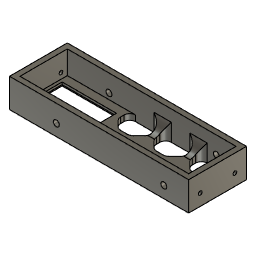
Grill_MAINS_Panels (Autodesk Fusion 360 design; units mm, degrees)
Autodesk Fusion 360 part; units mm, degrees
sketch "Skizze1" plane through (0, 0, 0) normal (0, 0, 1) x (1, 0, 0)
  line L0 (0, 0) -> (155, 0)
  line L1 (155, 0) -> (155, 50)
  line L2 (155, 50) -> (0, 50)
  line L3 (0, 50) -> (0, 0)
  dimension "d1" = 155
  dimension "d2" = 50
  constraint horizontal L0
  constraint vertical L1
  constraint horizontal L2
  constraint vertical L3
  constraint coincident L0.start L3.end
  measures "d1" distance of L0.start L0.end
  measures "d2" distance of L0.start L2.end
extrude "Extrusion1" add sketch "Skizze1" along normal blind 5
sketch "Skizze2" plane through (0, 0, 5) normal (0, 0, 1) x (-1, 0, 0)
  line L0 (0, -50) -> (0, 0)
  line L1 (0, 0) -> (-155, 0)
  line L2 (-155, 0) -> (-155, -50)
  line L3 (-155, -50) -> (0, -50)
  line L4 (-4.5, -45.5) -> (-150.5, -45.5)
  line L5 (-150.5, -45.5) -> (-150.5, -4.5)
  line L6 (-150.5, -4.5) -> (-4.5, -4.5)
  line L7 (-4.5, -4.5) -> (-4.5, -45.5)
  constraint horizontal L4
  constraint vertical L5
  constraint horizontal L6
  constraint vertical L7
extrude "Extrusion2" add sketch "Skizze2" along normal blind 20
sketch "Skizze3" plane through (0, 0, 5) normal (0, 0, 1) x (-1, 0, 0)
  line L0 (-150.5, -4.5) -> (-150.5, -45.5)
  line L1 (-4.5, -45.5) -> (-4.5, -4.5)
  line L2 (-4.5, -22.5) -> (-14.5, -22.5)
  line L3 (-4.5, -27.5) -> (-14.5, -27.5)
  line L4 (-22.5, -45.5) -> (-22.5, -35.5)
  line L5 (-22.5, -4.5) -> (-22.5, -14.5)
  line L6 (-14.5, -22.5) -> (-22.5, -14.5)
  line L7 (-14.5, -27.5) -> (-22.5, -35.5)
  line L8 (-22.5, -4.5) -> (-27.5, -4.5)
  line L9 (-27.5, -45.5) -> (-27.5, -35.5)
  line L10 (-27.5, -4.5) -> (-27.5, -14.5)
  line L11 (-27.5, -4.5) -> (-35.5, -4.5)
  line L12 (-35.5, -4.5) -> (-35.5, -22.5)
  line L13 (-27.5, -35.5) -> (-35.5, -27.5)
  line L14 (-27.5, -14.5) -> (-35.5, -22.5)
  line L15 (-35.5, -22.5) -> (-45.5, -22.5)
  line L16 (-35.5, -27.5) -> (-45.5, -27.5)
  line L17 (-35.5, -4.5) -> (-53.5, -4.5)
  line L18 (-53.5, -4.5) -> (-53.5, -14.5)
  line L19 (-45.5, -22.5) -> (-53.5, -14.5)
  line L20 (-53.5, -45.5) -> (-53.5, -35.5)
  line L21 (-53.5, -35.5) -> (-45.5, -27.5)
  line L22 (-53.5, -45.5) -> (-58.5, -45.5)
  line L23 (-58.5, -45.5) -> (-58.5, -35.5)
  line L24 (-53.5, -4.5) -> (-58.5, -4.5)
  line L25 (-58.5, -4.5) -> (-58.5, -14.5)
  line L26 (-58.5, -4.5) -> (-66.5, -4.5)
  line L27 (-66.5, -4.5) -> (-66.5, -22.5)
  line L28 (-58.5, -14.5) -> (-66.5, -22.5)
  line L29 (-66.5, -27.5) -> (-58.5, -35.5)
  line L30 (-66.5, -27.5) -> (-76.5, -27.5)
  line L31 (-66.5, -22.5) -> (-76.5, -22.5)
  line L32 (-76.5, -4.5) -> (-84.5, -4.5)
  line L33 (-84.5, -4.5) -> (-84.5, -14.5)
  line L34 (-84.5, -14.5) -> (-76.5, -22.5)
  line L35 (-76.5, -27.5) -> (-84.5, -35.5)
  line L36 (-84.5, -35.5) -> (-84.5, -45.5)
  line L37 (-84.5, -45.5) -> (-89.5, -45.5)
  line L38 (-89.5, -45.5) -> (-89.5, -35.5)
  line L39 (-89.5, -35.5) -> (-97.5, -27.5)
  line L40 (-89.5, -35.5) -> (-78.1863, -35.5) construction
  line L41 (-97.5, -27.5) -> (-107.5, -27.5)
  line L42 (-107.5, -27.5) -> (-115.5, -35.5)
  line L43 (-115.5, -35.5) -> (-115.5, -45.5)
  line L44 (-84.5, -4.5) -> (-89.5, -4.5)
  line L45 (-89.5, -4.5) -> (-89.5, -14.5)
  line L46 (-89.5, -14.5) -> (-97.5, -22.5)
  line L47 (-89.5, -14.5) -> (-78.1863, -14.5) construction
  line L48 (-97.5, -22.5) -> (-107.5, -22.5)
  line L49 (-107.5, -22.5) -> (-115.5, -14.5)
  line L50 (-115.5, -14.5) -> (-115.5, -4.5)
  line L51 (-115.5, -4.5) -> (-120.5, -4.5)
  line L52 (-120.5, -4.5) -> (-120.5, -14.5)
  line L53 (-120.5, -14.5) -> (-128.5, -22.5)
  line L54 (-120.5, -14.5) -> (-109.1863, -14.5) construction
  line L55 (-128.5, -22.5) -> (-138.5, -22.5)
  line L56 (-138.5, -22.5) -> (-146.5, -14.5)
  line L57 (-138.5, -22.5) -> (-127.1863, -22.5) construction
  line L58 (-146.5, -14.5) -> (-146.5, -4.5)
  line L59 (-138.5, -27.5) -> (-146.5, -35.5)
  line L60 (-146.5, -35.5) -> (-146.5, -45.5)
  line L61 (-138.5, -27.5) -> (-128.5, -27.5)
  line L62 (-128.5, -27.5) -> (-120.5, -35.5)
  line L63 (-128.5, -27.5) -> (-117.1863, -27.5) construction
  line L64 (-120.5, -35.5) -> (-120.5, -45.5)
  line L65 (-4.5, -27.5) -> (-4.5, -45.5)
  line L66 (-4.5, -45.5) -> (-22.5, -45.5)
  line L67 (-4.5, -22.5) -> (-4.5, -4.5)
  line L68 (-4.5, -4.5) -> (-22.5, -4.5)
  line L69 (-27.5, -4.5) -> (-53.5, -4.5)
  line L70 (-58.5, -4.5) -> (-84.5, -4.5)
  line L71 (-89.5, -4.5) -> (-115.5, -4.5)
  line L72 (-120.5, -4.5) -> (-146.5, -4.5)
  line L73 (-146.5, -45.5) -> (-120.5, -45.5)
  line L74 (-115.5, -45.5) -> (-89.5, -45.5)
  line L75 (-84.5, -45.5) -> (-58.5, -45.5)
  line L76 (-53.5, -45.5) -> (-27.5, -45.5)
  dimension "d13" = 10
  dimension "d14" = 10
  dimension "d15" = 18
  dimension "d16" = 10
  dimension "d17" = 18
  dimension "d18" = 10
  dimension "d19" = 5
  dimension "d20" = 5
  dimension "d21" = 10
  dimension "d22" = 10
  dimension "d23" = 8
  dimension "d24" = 18
  dimension "d25" = 5
  dimension "d26" = 10
  dimension "d27" = 10
  dimension "d28" = 18
  dimension "d29" = 10
  dimension "d30" = 10
  dimension "d31" = 5
  dimension "d32" = 10
  dimension "d33" = 5
  dimension "d34" = 10
  dimension "d35" = 8
  dimension "d36" = 18
  dimension "d37" = 5
  dimension "d38" = 10
  dimension "d39" = 10
  dimension "d40" = 8
  dimension "d41" = 10
  dimension "d42" = 5
  dimension "d43" = 10
  dimension "d44" = 135
  dimension "d45" = 10
  dimension "d46" = 5
  dimension "d47" = 10
  dimension "d48" = 135
  dimension "d49" = 10
  dimension "d50" = 5
  dimension "d51" = 10
  dimension "d52" = 135
  dimension "d53" = 10
  dimension "d54" = 135
  dimension "d56" = 10
  dimension "d57" = 45
  constraint perpendicular L1 L3
  constraint perpendicular L5 L8
  constraint perpendicular L8 L10
  constraint perpendicular L10 L11
  constraint perpendicular L11 L12
  constraint perpendicular L12 L17
  constraint perpendicular L17 L18
  constraint perpendicular L20 L22
  constraint perpendicular L18 L24
  constraint perpendicular L24 L25
  constraint perpendicular L25 L26
  constraint perpendicular L26 L27
  constraint perpendicular L28 L29
  constraint perpendicular L27 L31
  constraint perpendicular L32 L33
  constraint perpendicular L34 L35
  constraint perpendicular L36 L37
  constraint perpendicular L37 L38
  constraint horizontal L40
  constraint perpendicular L38 L41
  constraint perpendicular L39 L42
  constraint perpendicular L33 L44
  constraint perpendicular L44 L45
  constraint horizontal L47
  constraint perpendicular L46 L49
  constraint perpendicular L50 L51
  constraint horizontal L54
  constraint horizontal L57
  constraint horizontal L63
  constraint coincident L1.start L65.end
  constraint perpendicular L3 L65
  constraint perpendicular L65 L66
  constraint coincident L1.end L67.end
  constraint perpendicular L2 L67
  constraint perpendicular L5 L68
  constraint perpendicular L33 L70
  constraint perpendicular L50 L71
  constraint perpendicular L58 L72
  constraint perpendicular L64 L73
  constraint perpendicular L38 L74
  constraint perpendicular L23 L75
  constraint perpendicular L9 L76
  measures "d13" distance of L2.start L2.end
  measures "d14" distance of L3.start L3.end
  measures "d15" distance of L1.start L4.start
  measures "d16" distance of L4.start L4.end
  measures "d17" distance of L1.end L5.start
  measures "d18" distance of L5.start L5.end
  measures "d19" distance of L4.start L9.start
  measures "d20" distance of L5.start L8.end
  measures "d21" distance of L9.start L9.end
  measures "d22" distance of L8.end L10.end
  measures "d23" distance of L8.end L11.end
  measures "d24" distance of L11.end L12.end
  measures "d25" distance of L12.end L13.end
  measures "d26" distance of L12.end L15.end
  measures "d27" distance of L13.end L16.end
  measures "d28" distance of L11.end L17.end
  measures "d29" distance of L17.end L18.end
  measures "d30" distance of L20.start L20.end
  measures "d31" distance of L20.start L22.end
  measures "d32" distance of L22.end L23.end
  measures "d33" distance of L17.end L24.end
  measures "d34" distance of L24.end L25.end
  measures "d35" distance of L24.end L26.end
  measures "d36" distance of L26.end L27.end
  measures "d37" distance of L27.end L29.start
  measures "d38" distance of L29.start L30.end
  measures "d39" distance of L27.end L31.end
  measures "d40" distance of L32.start L32.end
  measures "d41" distance of L32.end L33.end
  measures "d42" distance of L36.end L37.end
  measures "d43" distance of L37.end L38.end
  measures "d44" angle of L39 L40
  measures "d45" distance of L39.end L41.end
  measures "d46" distance of L32.end L44.end
  measures "d47" distance of L44.end L45.end
  measures "d48" angle of L46 L47
  measures "d49" distance of L46.end L48.end
  measures "d50" distance of L50.end L51.end
  measures "d51" distance of L51.end L52.end
  measures "d52" angle of L53 L54
  measures "d53" distance of L53.end L55.end
  measures "d54" angle of L56 L57
  measures "d56" distance of L59.start L61.end
  measures "d57" angle of L62 L63
extrude "Extrusion3" cut sketch "Skizze3" against normal blind 5
fillet "Abrundung1" radius 5 56 edges at (22.5, 45.5, 2.5) (53.5, 45.5, 2.5) (84.5, 45.5, 2.5) (115.5, 45.5, 2.5) (146.5, 45.5, 2.5) (146.5, 35.5, 2.5) (120.5, 35.5, 2.5) (128.5, 27.5, 2.5) (138.5, 27.5, 2.5) (115.5, 35.5, 2.5) (107.5, 27.5, 2.5) (97.5, 27.5, 2.5) (89.5, 35.5, 2.5) (89.5, 45.5, 2.5) (120.5, 45.5, 2.5) (146.5, 14.5, 2.5) (138.5, 22.5, 2.5) (128.5, 22.5, 2.5) (120.5, 14.5, 2.5) (115.5, 14.5, 2.5) (107.5, 22.5, 2.5) (97.5, 22.5, 2.5) (89.5, 14.5, 2.5) (84.5, 35.5, 2.5) (84.5, 14.5, 2.5) (76.5, 22.5, 2.5) (76.5, 27.5, 2.5) (66.5, 27.5, 2.5) (66.5, 22.5, 2.5) (58.5, 14.5, 2.5) (58.5, 35.5, 2.5) (58.5, 45.5, 2.5) (53.5, 35.5, 2.5) (45.5, 27.5, 2.5) (45.5, 22.5, 2.5) (53.5, 14.5, 2.5) (35.5, 27.5, 2.5) (35.5, 22.5, 2.5) (27.5, 14.5, 2.5) (27.5, 35.5, 2.5) (27.5, 45.5, 2.5) (22.5, 35.5, 2.5) (14.5, 27.5, 2.5) (14.5, 22.5, 2.5) (22.5, 14.5, 2.5) (146.5, 4.5, 2.5) (120.5, 4.5, 2.5) (115.5, 4.5, 2.5) (84.5, 4.5, 2.5) (89.5, 4.5, 2.5) (58.5, 4.5, 2.5) (53.5, 4.5, 2.5) (27.5, 4.5, 2.5) (22.5, 4.5, 2.5) (4.5, 22.5, 2.5) (4.5, 27.5, 2.5)
fillet "Abrundung2" radius 10 5 edges at (25, 45.5, 5) (56, 45.5, 5) (87, 45.5, 5) (118, 45.5, 5) (146, 45.5, 5)
fillet "Abrundung3" radius 10 5 edges at (146, 4.5, 5) (118, 4.5, 5) (87, 4.5, 5) (56, 4.5, 5) (25, 4.5, 5)
extrude "Extrusion4" cut 1 faces at (53.1667, 48.5, 25) along direction (0, 0, -1) blind 5
hole "Bohrung1" at (0, 40, 10) direction (1, 0, 0) diameter 3.2 depth 10 tip angle 180
hole "Bohrung2" at (0, 10, 10) direction (1, 0, 0) diameter 3.2 depth 10 tip angle 180
hole "Bohrung3" at (40.5, 45.5, 10) direction (0, 1, 0) diameter 5.2 depth 10 tip angle 180
hole "Bohrung4" at (133.5, 45.5, 10) direction (0, 1, 0) diameter 5.2 depth 10 tip angle 180
hole "Bohrung5" at (133.5, 4.5, 10) direction (0, -1, 0) diameter 5.2 depth 10 tip angle 180
hole "Bohrung6" at (40.5, 4.5, 10) direction (0, -1, 0) diameter 5.2 depth 10 tip angle 180
delete_face "Fläche löschen1" 1 faces at (9.2621, 27.5057, 3.3333)
delete_face "Fläche löschen2" 1 faces at (9.2621, 22.4943, 3.3333)
delete_face "Fläche löschen3" 1 faces at (23.4001, 5.0158, 11.8299)
delete_face "Fläche löschen4" 1 faces at (26.8017, 45.2968, 12.9942)
sketch "Skizze4" plane through (0, 0, 5) normal (0, 0, 1) x (-1, 0, 0)
  line L0 (-22.5, -40.5) -> (-22.5, -37.5711)
  arc A0 (-21.0355, -34.0355) -> (-22.5, -37.5711) centre (-17.5, -37.5711) ccw
  line L1 (-21.0355, -34.0355) -> (-15.9645, -28.9645)
  arc A1 (-12.4289, -27.5) -> (-15.9645, -28.9645) centre (-12.4289, -32.5) ccw
  line L2 (-12.4289, -27.5) -> (-4.5, -27.5)
  line L3 (-4.5, -27.5) -> (-4.5, -22.5)
  line L4 (-4.5, -22.5) -> (-12.4289, -22.5)
  arc A2 (-15.9645, -21.0355) -> (-12.4289, -22.5) centre (-12.4289, -17.5) ccw
  line L5 (-15.9645, -21.0355) -> (-21.0355, -15.9645)
  arc A3 (-22.5, -12.4289) -> (-21.0355, -15.9645) centre (-17.5, -12.4289) ccw
  line L6 (-22.5, -12.4289) -> (-22.5, -9.5)
  arc A4 (-17.5, -4.5) -> (-22.5, -9.5) centre (-17.5, -9.5) ccw
  line L7 (-17.5, -4.5) -> (-32.5, -4.5)
  arc A5 (-27.5, -9.5) -> (-32.5, -4.5) centre (-32.5, -9.5) ccw
  line L8 (-27.5, -9.5) -> (-27.5, -12.4289)
  arc A6 (-28.9645, -15.9645) -> (-27.5, -12.4289) centre (-32.5, -12.4289) ccw
  line L9 (-28.9645, -15.9645) -> (-34.0355, -21.0355)
  arc A7 (-37.5711, -22.5) -> (-34.0355, -21.0355) centre (-37.5711, -17.5) ccw
  line L10 (-37.5711, -22.5) -> (-43.4289, -22.5)
  arc A8 (-46.9645, -21.0355) -> (-43.4289, -22.5) centre (-43.4289, -17.5) ccw
  line L11 (-46.9645, -21.0355) -> (-52.0355, -15.9645)
  arc A9 (-53.0509, -14.5) -> (-52.0355, -15.9645) centre (-48.5, -12.4289) ccw
  line L12 (-53.0509, -14.5) -> (-58.9491, -14.5)
  arc A10 (-59.9645, -15.9645) -> (-58.9491, -14.5) centre (-63.5, -12.4289) ccw
  line L13 (-59.9645, -15.9645) -> (-65.0355, -21.0355)
  arc A11 (-68.5711, -22.5) -> (-65.0355, -21.0355) centre (-68.5711, -17.5) ccw
  line L14 (-68.5711, -22.5) -> (-74.4289, -22.5)
  arc A12 (-77.9645, -21.0355) -> (-74.4289, -22.5) centre (-74.4289, -17.5) ccw
  line L15 (-77.9645, -21.0355) -> (-83.0355, -15.9645)
  arc A13 (-84.0509, -14.5) -> (-83.0355, -15.9645) centre (-79.5, -12.4289) ccw
  line L16 (-84.0509, -14.5) -> (-89.9491, -14.5)
  arc A14 (-90.9645, -15.9645) -> (-89.9491, -14.5) centre (-94.5, -12.4289) ccw
  line L17 (-90.9645, -15.9645) -> (-96.0355, -21.0355)
  arc A15 (-99.5711, -22.5) -> (-96.0355, -21.0355) centre (-99.5711, -17.5) ccw
  line L18 (-99.5711, -22.5) -> (-105.4289, -22.5)
  arc A16 (-108.9645, -21.0355) -> (-105.4289, -22.5) centre (-105.4289, -17.5) ccw
  line L19 (-108.9645, -21.0355) -> (-114.0355, -15.9645)
  arc A17 (-115.0509, -14.5) -> (-114.0355, -15.9645) centre (-110.5, -12.4289) ccw
  line L20 (-115.0509, -14.5) -> (-120.9491, -14.5)
  arc A18 (-121.9645, -15.9645) -> (-120.9491, -14.5) centre (-125.5, -12.4289) ccw
  line L21 (-121.9645, -15.9645) -> (-127.0355, -21.0355)
  arc A19 (-130.5711, -22.5) -> (-127.0355, -21.0355) centre (-130.5711, -17.5) ccw
  line L22 (-130.5711, -22.5) -> (-136.4289, -22.5)
  arc A20 (-139.9645, -21.0355) -> (-136.4289, -22.5) centre (-136.4289, -17.5) ccw
  line L23 (-139.9645, -21.0355) -> (-145.0355, -15.9645)
  arc A21 (-146.0509, -14.5) -> (-145.0355, -15.9645) centre (-141.5, -12.4289) ccw
  line L24 (-146.0509, -14.5) -> (-150.5, -14.5)
  line L25 (-150.5, -14.5) -> (-150.5, -35.5)
  line L26 (-150.5, -35.5) -> (-146.0509, -35.5)
  arc A22 (-145.0355, -34.0355) -> (-146.0509, -35.5) centre (-141.5, -37.5711) ccw
  line L27 (-145.0355, -34.0355) -> (-139.9645, -28.9645)
  arc A23 (-136.4289, -27.5) -> (-139.9645, -28.9645) centre (-136.4289, -32.5) ccw
  line L28 (-136.4289, -27.5) -> (-130.5711, -27.5)
  arc A24 (-127.0355, -28.9645) -> (-130.5711, -27.5) centre (-130.5711, -32.5) ccw
  line L29 (-127.0355, -28.9645) -> (-121.9645, -34.0355)
  arc A25 (-120.9491, -35.5) -> (-121.9645, -34.0355) centre (-125.5, -37.5711) ccw
  line L30 (-120.9491, -35.5) -> (-115.0509, -35.5)
  arc A26 (-114.0355, -34.0355) -> (-115.0509, -35.5) centre (-110.5, -37.5711) ccw
  line L31 (-114.0355, -34.0355) -> (-108.9645, -28.9645)
  arc A27 (-105.4289, -27.5) -> (-108.9645, -28.9645) centre (-105.4289, -32.5) ccw
  line L32 (-105.4289, -27.5) -> (-99.5711, -27.5)
  arc A28 (-96.0355, -28.9645) -> (-99.5711, -27.5) centre (-99.5711, -32.5) ccw
  line L33 (-96.0355, -28.9645) -> (-90.9645, -34.0355)
  arc A29 (-89.9491, -35.5) -> (-90.9645, -34.0355) centre (-94.5, -37.5711) ccw
  line L34 (-89.9491, -35.5) -> (-84.0509, -35.5)
  arc A30 (-83.0355, -34.0355) -> (-84.0509, -35.5) centre (-79.5, -37.5711) ccw
  line L35 (-83.0355, -34.0355) -> (-77.9645, -28.9645)
  arc A31 (-74.4289, -27.5) -> (-77.9645, -28.9645) centre (-74.4289, -32.5) ccw
  line L36 (-74.4289, -27.5) -> (-68.5711, -27.5)
  arc A32 (-65.0355, -28.9645) -> (-68.5711, -27.5) centre (-68.5711, -32.5) ccw
  line L37 (-65.0355, -28.9645) -> (-59.9645, -34.0355)
  arc A33 (-58.9491, -35.5) -> (-59.9645, -34.0355) centre (-63.5, -37.5711) ccw
  line L38 (-58.9491, -35.5) -> (-53.0509, -35.5)
  arc A34 (-52.0355, -34.0355) -> (-53.0509, -35.5) centre (-48.5, -37.5711) ccw
  line L39 (-52.0355, -34.0355) -> (-46.9645, -28.9645)
  arc A35 (-43.4289, -27.5) -> (-46.9645, -28.9645) centre (-43.4289, -32.5) ccw
  line L40 (-43.4289, -27.5) -> (-37.5711, -27.5)
  arc A36 (-34.0355, -28.9645) -> (-37.5711, -27.5) centre (-37.5711, -32.5) ccw
  line L41 (-34.0355, -28.9645) -> (-28.9645, -34.0355)
  arc A37 (-27.5, -37.5711) -> (-28.9645, -34.0355) centre (-32.5, -37.5711) ccw
  line L42 (-27.5, -37.5711) -> (-27.5, -40.5)
  arc A38 (-32.5, -45.5) -> (-27.5, -40.5) centre (-32.5, -40.5) ccw
  line L43 (-32.5, -45.5) -> (-17.5, -45.5)
  arc A39 (-22.5, -40.5) -> (-17.5, -45.5) centre (-17.5, -40.5) ccw
  line L44 (-4.5, -25) -> (-4.5, -45.5)
  line L45 (-4.5, -45.5) -> (-45.5, -45.5)
  line L46 (-45.5, -45.5) -> (-45.5, -4.5)
  line L47 (-45.5, -4.5) -> (-4.5, -4.5)
  line L48 (-4.5, -4.5) -> (-4.5, -45.5)
  dimension "d98" = 20.5
  dimension "d99" = 41
  dimension "d100" = 41
  constraint midpoint L3 L44.start
  constraint perpendicular L2 L44
  constraint horizontal L45
  constraint vertical L46
  constraint horizontal L47
  constraint vertical L48
  measures "d98" distance of L44.start L44.end
  measures "d99" distance of L44.end L45.end
  measures "d100" distance of L44.end L47.end
extrude "Extrusion5" add sketch "Skizze4" against normal blind 5 contours L0 A0 L1 A1 L2 A39 L44 L45 L48 | A35 L40 A36 L41 A37 L42 A38 L45 L46 | A5 L8 A6 L9 A7 L10 A8 L46 L47 | L4 A2 L5 A3 L6 A4 L47 L48
hole "Bohrung7" at (9, 41, 5) direction (0, 0, -1) diameter 3.2 depth 10 tip angle 180
hole "Bohrung8" at (9, 9, 5) direction (0, 0, -1) diameter 3.2 depth 10 tip angle 180
hole "Bohrung9" at (41, 41, 5) direction (0, 0, -1) diameter 3.2 depth 10 tip angle 180
hole "Bohrung10" at (41, 9, 5) direction (0, 0, -1) diameter 3.2 depth 10 tip angle 180
sketch "Skizze5" plane through (0, 0, 5) normal (0, 0, 1) x (-1, 0, 0)
  circle A0 centre (-41, -9) radius 1.6
  circle A1 centre (-41, -41) radius 1.6
  circle A2 centre (-9, -9) radius 1.6
  circle A3 centre (-9, -41) radius 1.6
  line L0 (-45.5, -45.5) -> (-4.5, -45.5)
  line L1 (-4.5, -45.5) -> (-4.5, -4.5)
  line L2 (-4.5, -4.5) -> (-45.5, -4.5)
  line L3 (-45.5, -4.5) -> (-45.5, -22.0509)
  arc A4 (-46.9645, -21.0355) -> (-45.5, -22.0509) centre (-43.4289, -17.5) ccw
  line L4 (-46.9645, -21.0355) -> (-52.0355, -15.9645)
  arc A5 (-53.0509, -14.5) -> (-52.0355, -15.9645) centre (-48.5, -12.4289) ccw
  line L5 (-53.0509, -14.5) -> (-58.9491, -14.5)
  arc A6 (-59.9645, -15.9645) -> (-58.9491, -14.5) centre (-63.5, -12.4289) ccw
  line L6 (-59.9645, -15.9645) -> (-65.0355, -21.0355)
  arc A7 (-68.5711, -22.5) -> (-65.0355, -21.0355) centre (-68.5711, -17.5) ccw
  line L7 (-68.5711, -22.5) -> (-74.4289, -22.5)
  arc A8 (-77.9645, -21.0355) -> (-74.4289, -22.5) centre (-74.4289, -17.5) ccw
  line L8 (-77.9645, -21.0355) -> (-83.0355, -15.9645)
  arc A9 (-84.0509, -14.5) -> (-83.0355, -15.9645) centre (-79.5, -12.4289) ccw
  line L9 (-84.0509, -14.5) -> (-89.9491, -14.5)
  arc A10 (-90.9645, -15.9645) -> (-89.9491, -14.5) centre (-94.5, -12.4289) ccw
  line L10 (-90.9645, -15.9645) -> (-96.0355, -21.0355)
  arc A11 (-99.5711, -22.5) -> (-96.0355, -21.0355) centre (-99.5711, -17.5) ccw
  line L11 (-99.5711, -22.5) -> (-105.4289, -22.5)
  arc A12 (-108.9645, -21.0355) -> (-105.4289, -22.5) centre (-105.4289, -17.5) ccw
  line L12 (-108.9645, -21.0355) -> (-114.0355, -15.9645)
  arc A13 (-115.0509, -14.5) -> (-114.0355, -15.9645) centre (-110.5, -12.4289) ccw
  line L13 (-115.0509, -14.5) -> (-120.9491, -14.5)
  arc A14 (-121.9645, -15.9645) -> (-120.9491, -14.5) centre (-125.5, -12.4289) ccw
  line L14 (-121.9645, -15.9645) -> (-127.0355, -21.0355)
  arc A15 (-130.5711, -22.5) -> (-127.0355, -21.0355) centre (-130.5711, -17.5) ccw
  line L15 (-130.5711, -22.5) -> (-136.4289, -22.5)
  arc A16 (-139.9645, -21.0355) -> (-136.4289, -22.5) centre (-136.4289, -17.5) ccw
  line L16 (-139.9645, -21.0355) -> (-145.0355, -15.9645)
  arc A17 (-146.0509, -14.5) -> (-145.0355, -15.9645) centre (-141.5, -12.4289) ccw
  line L17 (-146.0509, -14.5) -> (-150.5, -14.5)
  line L18 (-150.5, -14.5) -> (-150.5, -35.5)
  line L19 (-150.5, -35.5) -> (-146.0509, -35.5)
  arc A18 (-145.0355, -34.0355) -> (-146.0509, -35.5) centre (-141.5, -37.5711) ccw
  line L20 (-145.0355, -34.0355) -> (-139.9645, -28.9645)
  arc A19 (-136.4289, -27.5) -> (-139.9645, -28.9645) centre (-136.4289, -32.5) ccw
  line L21 (-136.4289, -27.5) -> (-130.5711, -27.5)
  arc A20 (-127.0355, -28.9645) -> (-130.5711, -27.5) centre (-130.5711, -32.5) ccw
  line L22 (-127.0355, -28.9645) -> (-121.9645, -34.0355)
  arc A21 (-120.9491, -35.5) -> (-121.9645, -34.0355) centre (-125.5, -37.5711) ccw
  line L23 (-120.9491, -35.5) -> (-115.0509, -35.5)
  arc A22 (-114.0355, -34.0355) -> (-115.0509, -35.5) centre (-110.5, -37.5711) ccw
  line L24 (-114.0355, -34.0355) -> (-108.9645, -28.9645)
  arc A23 (-105.4289, -27.5) -> (-108.9645, -28.9645) centre (-105.4289, -32.5) ccw
  line L25 (-105.4289, -27.5) -> (-99.5711, -27.5)
  arc A24 (-96.0355, -28.9645) -> (-99.5711, -27.5) centre (-99.5711, -32.5) ccw
  line L26 (-96.0355, -28.9645) -> (-90.9645, -34.0355)
  arc A25 (-89.9491, -35.5) -> (-90.9645, -34.0355) centre (-94.5, -37.5711) ccw
  line L27 (-89.9491, -35.5) -> (-84.0509, -35.5)
  arc A26 (-83.0355, -34.0355) -> (-84.0509, -35.5) centre (-79.5, -37.5711) ccw
  line L28 (-83.0355, -34.0355) -> (-77.9645, -28.9645)
  arc A27 (-74.4289, -27.5) -> (-77.9645, -28.9645) centre (-74.4289, -32.5) ccw
  line L29 (-74.4289, -27.5) -> (-68.5711, -27.5)
  arc A28 (-65.0355, -28.9645) -> (-68.5711, -27.5) centre (-68.5711, -32.5) ccw
  line L30 (-65.0355, -28.9645) -> (-59.9645, -34.0355)
  arc A29 (-58.9491, -35.5) -> (-59.9645, -34.0355) centre (-63.5, -37.5711) ccw
  line L31 (-58.9491, -35.5) -> (-53.0509, -35.5)
  arc A30 (-52.0355, -34.0355) -> (-53.0509, -35.5) centre (-48.5, -37.5711) ccw
  line L32 (-52.0355, -34.0355) -> (-46.9645, -28.9645)
  arc A31 (-45.5, -27.9491) -> (-46.9645, -28.9645) centre (-43.4289, -32.5) ccw
  line L33 (-45.5, -27.9491) -> (-45.5, -45.5)
  circle A32 centre (-25, -25) radius 19
  dimension "d123" = 38
extrude "Extrusion6" cut sketch "Skizze5" against normal blind 5 contours A32
delete_face "Fläche löschen5" 1 faces at (54.1983, 45.2968, 12.9942)
delete_face "Fläche löschen6" 1 faces at (54.4001, 5.0158, 11.8299)
sketch "Skizze6" plane through (0, 0, 5) normal (0, 0, 1) x (-1, 0, 0)
  line L0 (-58.5, -9.5) -> (-58.5, -12.4289)
  arc A0 (-59.9645, -15.9645) -> (-58.5, -12.4289) centre (-63.5, -12.4289) ccw
  line L1 (-59.9645, -15.9645) -> (-65.0355, -21.0355)
  arc A1 (-68.5711, -22.5) -> (-65.0355, -21.0355) centre (-68.5711, -17.5) ccw
  line L2 (-68.5711, -22.5) -> (-74.4289, -22.5)
  arc A2 (-77.9645, -21.0355) -> (-74.4289, -22.5) centre (-74.4289, -17.5) ccw
  line L3 (-77.9645, -21.0355) -> (-83.0355, -15.9645)
  arc A3 (-84.0509, -14.5) -> (-83.0355, -15.9645) centre (-79.5, -12.4289) ccw
  line L4 (-84.0509, -14.5) -> (-89.9491, -14.5)
  arc A4 (-90.9645, -15.9645) -> (-89.9491, -14.5) centre (-94.5, -12.4289) ccw
  line L5 (-90.9645, -15.9645) -> (-96.0355, -21.0355)
  arc A5 (-99.5711, -22.5) -> (-96.0355, -21.0355) centre (-99.5711, -17.5) ccw
  line L6 (-99.5711, -22.5) -> (-105.4289, -22.5)
  arc A6 (-108.9645, -21.0355) -> (-105.4289, -22.5) centre (-105.4289, -17.5) ccw
  line L7 (-108.9645, -21.0355) -> (-114.0355, -15.9645)
  arc A7 (-115.0509, -14.5) -> (-114.0355, -15.9645) centre (-110.5, -12.4289) ccw
  line L8 (-115.0509, -14.5) -> (-120.9491, -14.5)
  arc A8 (-121.9645, -15.9645) -> (-120.9491, -14.5) centre (-125.5, -12.4289) ccw
  line L9 (-121.9645, -15.9645) -> (-127.0355, -21.0355)
  arc A9 (-130.5711, -22.5) -> (-127.0355, -21.0355) centre (-130.5711, -17.5) ccw
  line L10 (-130.5711, -22.5) -> (-136.4289, -22.5)
  arc A10 (-139.9645, -21.0355) -> (-136.4289, -22.5) centre (-136.4289, -17.5) ccw
  line L11 (-139.9645, -21.0355) -> (-145.0355, -15.9645)
  arc A11 (-146.0509, -14.5) -> (-145.0355, -15.9645) centre (-141.5, -12.4289) ccw
  line L12 (-146.0509, -14.5) -> (-150.5, -14.5)
  line L13 (-150.5, -14.5) -> (-150.5, -35.5)
  line L14 (-150.5, -35.5) -> (-146.0509, -35.5)
  arc A12 (-145.0355, -34.0355) -> (-146.0509, -35.5) centre (-141.5, -37.5711) ccw
  line L15 (-145.0355, -34.0355) -> (-139.9645, -28.9645)
  arc A13 (-136.4289, -27.5) -> (-139.9645, -28.9645) centre (-136.4289, -32.5) ccw
  line L16 (-136.4289, -27.5) -> (-130.5711, -27.5)
  arc A14 (-127.0355, -28.9645) -> (-130.5711, -27.5) centre (-130.5711, -32.5) ccw
  line L17 (-127.0355, -28.9645) -> (-121.9645, -34.0355)
  arc A15 (-120.9491, -35.5) -> (-121.9645, -34.0355) centre (-125.5, -37.5711) ccw
  line L18 (-120.9491, -35.5) -> (-115.0509, -35.5)
  arc A16 (-114.0355, -34.0355) -> (-115.0509, -35.5) centre (-110.5, -37.5711) ccw
  line L19 (-114.0355, -34.0355) -> (-108.9645, -28.9645)
  arc A17 (-105.4289, -27.5) -> (-108.9645, -28.9645) centre (-105.4289, -32.5) ccw
  line L20 (-105.4289, -27.5) -> (-99.5711, -27.5)
  arc A18 (-96.0355, -28.9645) -> (-99.5711, -27.5) centre (-99.5711, -32.5) ccw
  line L21 (-96.0355, -28.9645) -> (-90.9645, -34.0355)
  arc A19 (-89.9491, -35.5) -> (-90.9645, -34.0355) centre (-94.5, -37.5711) ccw
  line L22 (-89.9491, -35.5) -> (-84.0509, -35.5)
  arc A20 (-83.0355, -34.0355) -> (-84.0509, -35.5) centre (-79.5, -37.5711) ccw
  line L23 (-83.0355, -34.0355) -> (-77.9645, -28.9645)
  arc A21 (-74.4289, -27.5) -> (-77.9645, -28.9645) centre (-74.4289, -32.5) ccw
  line L24 (-74.4289, -27.5) -> (-68.5711, -27.5)
  arc A22 (-65.0355, -28.9645) -> (-68.5711, -27.5) centre (-68.5711, -32.5) ccw
  line L25 (-65.0355, -28.9645) -> (-59.9645, -34.0355)
  arc A23 (-58.5, -37.5711) -> (-59.9645, -34.0355) centre (-63.5, -37.5711) ccw
  line L26 (-58.5, -37.5711) -> (-58.5, -40.5)
  arc A24 (-63.5, -45.5) -> (-58.5, -40.5) centre (-63.5, -40.5) ccw
  line L27 (-63.5, -45.5) -> (-48.5, -45.5)
  arc A25 (-53.5, -40.5) -> (-48.5, -45.5) centre (-48.5, -40.5) ccw
  line L28 (-53.5, -40.5) -> (-53.5, -37.5711)
  arc A26 (-52.0355, -34.0355) -> (-53.5, -37.5711) centre (-48.5, -37.5711) ccw
  line L29 (-52.0355, -34.0355) -> (-46.9645, -28.9645)
  arc A27 (-45.5, -27.9491) -> (-46.9645, -28.9645) centre (-43.4289, -32.5) ccw
  line L30 (-45.5, -27.9491) -> (-45.5, -45.5)
  line L31 (-45.5, -45.5) -> (-4.5, -45.5)
  line L32 (-4.5, -45.5) -> (-4.5, -4.5)
  line L33 (-4.5, -4.5) -> (-45.5, -4.5)
  line L34 (-45.5, -4.5) -> (-45.5, -22.0509)
  arc A28 (-46.9645, -21.0355) -> (-45.5, -22.0509) centre (-43.4289, -17.5) ccw
  line L35 (-46.9645, -21.0355) -> (-52.0355, -15.9645)
  arc A29 (-53.5, -12.4289) -> (-52.0355, -15.9645) centre (-48.5, -12.4289) ccw
  line L36 (-53.5, -12.4289) -> (-53.5, -9.5)
  arc A30 (-48.5, -4.5) -> (-53.5, -9.5) centre (-48.5, -9.5) ccw
  line L37 (-48.5, -4.5) -> (-63.5, -4.5)
  arc A31 (-58.5, -9.5) -> (-63.5, -4.5) centre (-63.5, -9.5) ccw
  circle A32 centre (-25, -25) radius 19
  circle A33 centre (-41, -9) radius 1.6
  circle A34 centre (-41, -41) radius 1.6
  circle A35 centre (-9, -9) radius 1.6
  circle A36 centre (-9, -41) radius 1.6
  line L38 (-45.5, -45.5) -> (-55.5, -45.5)
  line L39 (-55.5, -45.5) -> (-55.5, -4.5)
  line L40 (-55.5, -4.5) -> (-45.5, -4.5)
  line L41 (-45.5, -4.5) -> (-45.5, -45.5)
  dimension "d126" = 10
  dimension "d127" = 41
  constraint horizontal L38
  constraint vertical L39
  constraint horizontal L40
  constraint vertical L41
  constraint coincident L30.end L31.start
  measures "d126" distance of L30.end L38.end
  measures "d127" distance of L30.end L33.end
extrude "Extrusion7" add sketch "Skizze6" against normal blind 5 contours L34 A28 L35 A29 L36 A30 L40 L41 | A25 L28 A26 L29 A27 L30 L38 L41
sketch "Skizze7" plane through (0, 0, 5) normal (0, 0, 1) x (-1, 0, 0)
  line L0 (-4.5, -4.5) -> (-63.5, -4.5)
  arc A0 (-58.5, -9.5) -> (-63.5, -4.5) centre (-63.5, -9.5) ccw
  line L1 (-58.5, -9.5) -> (-58.5, -12.4289)
  arc A1 (-59.9645, -15.9645) -> (-58.5, -12.4289) centre (-63.5, -12.4289) ccw
  line L2 (-59.9645, -15.9645) -> (-65.0355, -21.0355)
  arc A2 (-68.5711, -22.5) -> (-65.0355, -21.0355) centre (-68.5711, -17.5) ccw
  line L3 (-68.5711, -22.5) -> (-74.4289, -22.5)
  arc A3 (-77.9645, -21.0355) -> (-74.4289, -22.5) centre (-74.4289, -17.5) ccw
  line L4 (-77.9645, -21.0355) -> (-83.0355, -15.9645)
  arc A4 (-84.0509, -14.5) -> (-83.0355, -15.9645) centre (-79.5, -12.4289) ccw
  line L5 (-84.0509, -14.5) -> (-89.9491, -14.5)
  arc A5 (-90.9645, -15.9645) -> (-89.9491, -14.5) centre (-94.5, -12.4289) ccw
  line L6 (-90.9645, -15.9645) -> (-96.0355, -21.0355)
  arc A6 (-99.5711, -22.5) -> (-96.0355, -21.0355) centre (-99.5711, -17.5) ccw
  line L7 (-99.5711, -22.5) -> (-105.4289, -22.5)
  arc A7 (-108.9645, -21.0355) -> (-105.4289, -22.5) centre (-105.4289, -17.5) ccw
  line L8 (-108.9645, -21.0355) -> (-114.0355, -15.9645)
  arc A8 (-115.0509, -14.5) -> (-114.0355, -15.9645) centre (-110.5, -12.4289) ccw
  line L9 (-115.0509, -14.5) -> (-120.9491, -14.5)
  arc A9 (-121.9645, -15.9645) -> (-120.9491, -14.5) centre (-125.5, -12.4289) ccw
  line L10 (-121.9645, -15.9645) -> (-127.0355, -21.0355)
  arc A10 (-130.5711, -22.5) -> (-127.0355, -21.0355) centre (-130.5711, -17.5) ccw
  line L11 (-130.5711, -22.5) -> (-136.4289, -22.5)
  arc A11 (-139.9645, -21.0355) -> (-136.4289, -22.5) centre (-136.4289, -17.5) ccw
  line L12 (-139.9645, -21.0355) -> (-145.0355, -15.9645)
  arc A12 (-146.0509, -14.5) -> (-145.0355, -15.9645) centre (-141.5, -12.4289) ccw
  line L13 (-146.0509, -14.5) -> (-150.5, -14.5)
  line L14 (-150.5, -14.5) -> (-150.5, -35.5)
  line L15 (-150.5, -35.5) -> (-146.0509, -35.5)
  arc A13 (-145.0355, -34.0355) -> (-146.0509, -35.5) centre (-141.5, -37.5711) ccw
  line L16 (-145.0355, -34.0355) -> (-139.9645, -28.9645)
  arc A14 (-136.4289, -27.5) -> (-139.9645, -28.9645) centre (-136.4289, -32.5) ccw
  line L17 (-136.4289, -27.5) -> (-130.5711, -27.5)
  arc A15 (-127.0355, -28.9645) -> (-130.5711, -27.5) centre (-130.5711, -32.5) ccw
  line L18 (-127.0355, -28.9645) -> (-121.9645, -34.0355)
  arc A16 (-120.9491, -35.5) -> (-121.9645, -34.0355) centre (-125.5, -37.5711) ccw
  line L19 (-120.9491, -35.5) -> (-115.0509, -35.5)
  arc A17 (-114.0355, -34.0355) -> (-115.0509, -35.5) centre (-110.5, -37.5711) ccw
  line L20 (-114.0355, -34.0355) -> (-108.9645, -28.9645)
  arc A18 (-105.4289, -27.5) -> (-108.9645, -28.9645) centre (-105.4289, -32.5) ccw
  line L21 (-105.4289, -27.5) -> (-99.5711, -27.5)
  arc A19 (-96.0355, -28.9645) -> (-99.5711, -27.5) centre (-99.5711, -32.5) ccw
  line L22 (-96.0355, -28.9645) -> (-90.9645, -34.0355)
  arc A20 (-89.9491, -35.5) -> (-90.9645, -34.0355) centre (-94.5, -37.5711) ccw
  line L23 (-89.9491, -35.5) -> (-84.0509, -35.5)
  arc A21 (-83.0355, -34.0355) -> (-84.0509, -35.5) centre (-79.5, -37.5711) ccw
  line L24 (-83.0355, -34.0355) -> (-77.9645, -28.9645)
  arc A22 (-74.4289, -27.5) -> (-77.9645, -28.9645) centre (-74.4289, -32.5) ccw
  line L25 (-74.4289, -27.5) -> (-68.5711, -27.5)
  arc A23 (-65.0355, -28.9645) -> (-68.5711, -27.5) centre (-68.5711, -32.5) ccw
  line L26 (-65.0355, -28.9645) -> (-59.9645, -34.0355)
  arc A24 (-58.5, -37.5711) -> (-59.9645, -34.0355) centre (-63.5, -37.5711) ccw
  line L27 (-58.5, -37.5711) -> (-58.5, -40.5)
  arc A25 (-63.5, -45.5) -> (-58.5, -40.5) centre (-63.5, -40.5) ccw
  line L28 (-63.5, -45.5) -> (-4.5, -45.5)
  line L29 (-4.5, -45.5) -> (-4.5, -4.5)
  circle A26 centre (-25, -25) radius 19
  circle A27 centre (-41, -9) radius 1.6
  circle A28 centre (-41, -41) radius 1.6
  circle A29 centre (-9, -9) radius 1.6
  circle A30 centre (-9, -41) radius 1.6
  line L30 (-4.5, -45.5) -> (-50.3684, -45.5)
  line L31 (-50.3684, -45.5) -> (-50.3684, -4.5)
  line L32 (-50.3684, -4.5) -> (-4.5, -4.5)
  line L33 (-4.5, -4.5) -> (-4.5, -45.5)
  constraint horizontal L30
  constraint vertical L31
  constraint horizontal L32
  constraint vertical L33
  constraint coincident L0 L31.end
  constraint coincident L28.end L29.start
extrude "Extrusion8" add sketch "Skizze7" against normal blind 5 contours A26 | A27 | A28 | A29 | A30
hole "Bohrung11" at (155, 10, 10) direction (-1, 0, 0) diameter 3.2 depth 10 tip angle 180
hole "Bohrung12" at (155, 40, 10) direction (-1, 0, 0) diameter 3.2 depth 10 tip angle 180
sketch "Skizze8" plane through (0, 0, 5) normal (0, 0, 1) x (-1, 0, 0)
  line L0 (-4.5, -4.5) -> (-63.5, -4.5)
  arc A0 (-58.5, -9.5) -> (-63.5, -4.5) centre (-63.5, -9.5) ccw
  line L1 (-58.5, -9.5) -> (-58.5, -12.4289)
  arc A1 (-59.9645, -15.9645) -> (-58.5, -12.4289) centre (-63.5, -12.4289) ccw
  line L2 (-59.9645, -15.9645) -> (-65.0355, -21.0355)
  arc A2 (-68.5711, -22.5) -> (-65.0355, -21.0355) centre (-68.5711, -17.5) ccw
  line L3 (-68.5711, -22.5) -> (-74.4289, -22.5)
  arc A3 (-77.9645, -21.0355) -> (-74.4289, -22.5) centre (-74.4289, -17.5) ccw
  line L4 (-77.9645, -21.0355) -> (-83.0355, -15.9645)
  arc A4 (-84.0509, -14.5) -> (-83.0355, -15.9645) centre (-79.5, -12.4289) ccw
  line L5 (-84.0509, -14.5) -> (-89.9491, -14.5)
  arc A5 (-90.9645, -15.9645) -> (-89.9491, -14.5) centre (-94.5, -12.4289) ccw
  line L6 (-90.9645, -15.9645) -> (-96.0355, -21.0355)
  arc A6 (-99.5711, -22.5) -> (-96.0355, -21.0355) centre (-99.5711, -17.5) ccw
  line L7 (-99.5711, -22.5) -> (-105.4289, -22.5)
  arc A7 (-108.9645, -21.0355) -> (-105.4289, -22.5) centre (-105.4289, -17.5) ccw
  line L8 (-108.9645, -21.0355) -> (-114.0355, -15.9645)
  arc A8 (-115.0509, -14.5) -> (-114.0355, -15.9645) centre (-110.5, -12.4289) ccw
  line L9 (-115.0509, -14.5) -> (-120.9491, -14.5)
  arc A9 (-121.9645, -15.9645) -> (-120.9491, -14.5) centre (-125.5, -12.4289) ccw
  line L10 (-121.9645, -15.9645) -> (-127.0355, -21.0355)
  arc A10 (-130.5711, -22.5) -> (-127.0355, -21.0355) centre (-130.5711, -17.5) ccw
  line L11 (-130.5711, -22.5) -> (-136.4289, -22.5)
  arc A11 (-139.9645, -21.0355) -> (-136.4289, -22.5) centre (-136.4289, -17.5) ccw
  line L12 (-139.9645, -21.0355) -> (-145.0355, -15.9645)
  arc A12 (-146.0509, -14.5) -> (-145.0355, -15.9645) centre (-141.5, -12.4289) ccw
  line L13 (-146.0509, -14.5) -> (-150.5, -14.5)
  line L14 (-150.5, -14.5) -> (-150.5, -35.5)
  line L15 (-150.5, -35.5) -> (-146.0509, -35.5)
  arc A13 (-145.0355, -34.0355) -> (-146.0509, -35.5) centre (-141.5, -37.5711) ccw
  line L16 (-145.0355, -34.0355) -> (-139.9645, -28.9645)
  arc A14 (-136.4289, -27.5) -> (-139.9645, -28.9645) centre (-136.4289, -32.5) ccw
  line L17 (-136.4289, -27.5) -> (-130.5711, -27.5)
  arc A15 (-127.0355, -28.9645) -> (-130.5711, -27.5) centre (-130.5711, -32.5) ccw
  line L18 (-127.0355, -28.9645) -> (-121.9645, -34.0355)
  arc A16 (-120.9491, -35.5) -> (-121.9645, -34.0355) centre (-125.5, -37.5711) ccw
  line L19 (-120.9491, -35.5) -> (-115.0509, -35.5)
  arc A17 (-114.0355, -34.0355) -> (-115.0509, -35.5) centre (-110.5, -37.5711) ccw
  line L20 (-114.0355, -34.0355) -> (-108.9645, -28.9645)
  arc A18 (-105.4289, -27.5) -> (-108.9645, -28.9645) centre (-105.4289, -32.5) ccw
  line L21 (-105.4289, -27.5) -> (-99.5711, -27.5)
  arc A19 (-96.0355, -28.9645) -> (-99.5711, -27.5) centre (-99.5711, -32.5) ccw
  line L22 (-96.0355, -28.9645) -> (-90.9645, -34.0355)
  arc A20 (-89.9491, -35.5) -> (-90.9645, -34.0355) centre (-94.5, -37.5711) ccw
  line L23 (-89.9491, -35.5) -> (-84.0509, -35.5)
  arc A21 (-83.0355, -34.0355) -> (-84.0509, -35.5) centre (-79.5, -37.5711) ccw
  line L24 (-83.0355, -34.0355) -> (-77.9645, -28.9645)
  arc A22 (-74.4289, -27.5) -> (-77.9645, -28.9645) centre (-74.4289, -32.5) ccw
  line L25 (-74.4289, -27.5) -> (-68.5711, -27.5)
  arc A23 (-65.0355, -28.9645) -> (-68.5711, -27.5) centre (-68.5711, -32.5) ccw
  line L26 (-65.0355, -28.9645) -> (-59.9645, -34.0355)
  arc A24 (-58.5, -37.5711) -> (-59.9645, -34.0355) centre (-63.5, -37.5711) ccw
  line L27 (-58.5, -37.5711) -> (-58.5, -40.5)
  arc A25 (-63.5, -45.5) -> (-58.5, -40.5) centre (-63.5, -40.5) ccw
  line L28 (-63.5, -45.5) -> (-4.5, -45.5)
  line L29 (-4.5, -45.5) -> (-4.5, -4.5)
  line L30 (-4.5, -45.5) -> (-56.5, -45.5)
  line L31 (-56.5, -45.5) -> (-56.5, -4.5)
  line L32 (-56.5, -4.5) -> (-4.5, -4.5)
  line L33 (-4.5, -4.5) -> (-4.5, -45.5)
  line L34 (-54, -25) -> (-54, -38.5)
  line L35 (-54, -38.5) -> (-7, -38.5)
  line L36 (-7, -38.5) -> (-7, -11.5)
  line L37 (-7, -11.5) -> (-54, -11.5)
  line L38 (-54, -11.5) -> (-54, -25)
  dimension "d142" = 52
  dimension "d143" = 41
  dimension "d145" = 13.5
  dimension "d146" = 47
  dimension "d147" = 27
  dimension "d148" = 47
  constraint horizontal L30
  constraint vertical L31
  constraint horizontal L32
  constraint vertical L33
  constraint coincident L28.end L29.start
  constraint perpendicular L33 L35
  constraint perpendicular L35 L36
  constraint perpendicular L36 L37
  measures "d142" distance of L28.end L30.end
  measures "d143" distance of L28.end L0.start
  measures "d145" distance of L34.start L34.end
  measures "d146" distance of L34.end L35.end
  measures "d147" distance of L35.end L36.end
  measures "d148" distance of L36.end L37.end
extrude "Extrusion9" cut sketch "Skizze8" against normal blind 5 contours L34 L35 L36 L37 L38
sketch "Skizze9" plane through (0, 0, 0) normal (0, 0, -1) x (1, 0, 0)
  line L0 (54, -38.5) -> (7, -38.5)
  line L1 (7, -38.5) -> (7, -11.5)
  line L2 (7, -11.5) -> (54, -11.5)
  line L3 (54, -11.5) -> (54, -38.5)
  line L4 (0, 0) -> (0, -50)
  line L5 (0, -50) -> (155, -50)
  line L6 (155, -50) -> (155, 0)
  line L7 (155, 0) -> (0, 0)
  line L8 (94.5, -4.5) -> (110.5, -4.5)
  arc A0 (115.5, -9.5) -> (110.5, -4.5) centre (110.5, -9.5) ccw
  line L9 (115.5, -9.5) -> (115.5, -12.4289)
  arc A1 (114.0355, -15.9645) -> (115.5, -12.4289) centre (110.5, -12.4289) ccw
  line L10 (114.0355, -15.9645) -> (108.9645, -21.0355)
  arc A2 (105.4289, -22.5) -> (108.9645, -21.0355) centre (105.4289, -17.5) ccw
  line L11 (105.4289, -22.5) -> (99.5711, -22.5)
  arc A3 (96.0355, -21.0355) -> (99.5711, -22.5) centre (99.5711, -17.5) ccw
  line L12 (96.0355, -21.0355) -> (90.9645, -15.9645)
  arc A4 (89.5, -12.4289) -> (90.9645, -15.9645) centre (94.5, -12.4289) ccw
  line L13 (89.5, -12.4289) -> (89.5, -9.5)
  arc A5 (94.5, -4.5) -> (89.5, -9.5) centre (94.5, -9.5) ccw
  line L14 (63.5, -4.5) -> (79.5, -4.5)
  arc A6 (84.5, -9.5) -> (79.5, -4.5) centre (79.5, -9.5) ccw
  line L15 (84.5, -9.5) -> (84.5, -12.4289)
  arc A7 (83.0355, -15.9645) -> (84.5, -12.4289) centre (79.5, -12.4289) ccw
  line L16 (83.0355, -15.9645) -> (77.9645, -21.0355)
  arc A8 (74.4289, -22.5) -> (77.9645, -21.0355) centre (74.4289, -17.5) ccw
  line L17 (74.4289, -22.5) -> (68.5711, -22.5)
  arc A9 (65.0355, -21.0355) -> (68.5711, -22.5) centre (68.5711, -17.5) ccw
  line L18 (65.0355, -21.0355) -> (59.9645, -15.9645)
  arc A10 (58.5, -12.4289) -> (59.9645, -15.9645) centre (63.5, -12.4289) ccw
  line L19 (58.5, -12.4289) -> (58.5, -9.5)
  arc A11 (63.5, -4.5) -> (58.5, -9.5) centre (63.5, -9.5) ccw
  line L20 (146.5, -37.5711) -> (146.5, -40.5)
  arc A12 (141.5, -45.5) -> (146.5, -40.5) centre (141.5, -40.5) ccw
  line L21 (141.5, -45.5) -> (125.5, -45.5)
  arc A13 (120.5, -40.5) -> (125.5, -45.5) centre (125.5, -40.5) ccw
  line L22 (120.5, -40.5) -> (120.5, -37.5711)
  arc A14 (121.9645, -34.0355) -> (120.5, -37.5711) centre (125.5, -37.5711) ccw
  line L23 (121.9645, -34.0355) -> (127.0355, -28.9645)
  arc A15 (130.5711, -27.5) -> (127.0355, -28.9645) centre (130.5711, -32.5) ccw
  line L24 (130.5711, -27.5) -> (136.4289, -27.5)
  arc A16 (139.9645, -28.9645) -> (136.4289, -27.5) centre (136.4289, -32.5) ccw
  line L25 (139.9645, -28.9645) -> (145.0355, -34.0355)
  arc A17 (146.5, -37.5711) -> (145.0355, -34.0355) centre (141.5, -37.5711) ccw
  line L26 (89.5, -40.5) -> (89.5, -37.5711)
  arc A18 (90.9645, -34.0355) -> (89.5, -37.5711) centre (94.5, -37.5711) ccw
  line L27 (90.9645, -34.0355) -> (96.0355, -28.9645)
  arc A19 (99.5711, -27.5) -> (96.0355, -28.9645) centre (99.5711, -32.5) ccw
  line L28 (99.5711, -27.5) -> (105.4289, -27.5)
  arc A20 (108.9645, -28.9645) -> (105.4289, -27.5) centre (105.4289, -32.5) ccw
  line L29 (108.9645, -28.9645) -> (114.0355, -34.0355)
  arc A21 (115.5, -37.5711) -> (114.0355, -34.0355) centre (110.5, -37.5711) ccw
  line L30 (115.5, -37.5711) -> (115.5, -40.5)
  arc A22 (110.5, -45.5) -> (115.5, -40.5) centre (110.5, -40.5) ccw
  line L31 (110.5, -45.5) -> (94.5, -45.5)
  arc A23 (89.5, -40.5) -> (94.5, -45.5) centre (94.5, -40.5) ccw
  line L32 (77.9645, -28.9645) -> (83.0355, -34.0355)
  arc A24 (84.5, -37.5711) -> (83.0355, -34.0355) centre (79.5, -37.5711) ccw
  line L33 (84.5, -37.5711) -> (84.5, -40.5)
  arc A25 (79.5, -45.5) -> (84.5, -40.5) centre (79.5, -40.5) ccw
  line L34 (79.5, -45.5) -> (63.5, -45.5)
  arc A26 (58.5, -40.5) -> (63.5, -45.5) centre (63.5, -40.5) ccw
  line L35 (58.5, -40.5) -> (58.5, -37.5711)
  arc A27 (59.9645, -34.0355) -> (58.5, -37.5711) centre (63.5, -37.5711) ccw
  line L36 (59.9645, -34.0355) -> (65.0355, -28.9645)
  arc A28 (68.5711, -27.5) -> (65.0355, -28.9645) centre (68.5711, -32.5) ccw
  line L37 (68.5711, -27.5) -> (74.4289, -27.5)
  arc A29 (77.9645, -28.9645) -> (74.4289, -27.5) centre (74.4289, -32.5) ccw
  line L38 (125.5, -4.5) -> (141.5, -4.5)
  arc A30 (146.5, -9.5) -> (141.5, -4.5) centre (141.5, -9.5) ccw
  line L39 (146.5, -9.5) -> (146.5, -12.4289)
  arc A31 (145.0355, -15.9645) -> (146.5, -12.4289) centre (141.5, -12.4289) ccw
  line L40 (145.0355, -15.9645) -> (139.9645, -21.0355)
  arc A32 (136.4289, -22.5) -> (139.9645, -21.0355) centre (136.4289, -17.5) ccw
  line L41 (136.4289, -22.5) -> (130.5711, -22.5)
  arc A33 (127.0355, -21.0355) -> (130.5711, -22.5) centre (130.5711, -17.5) ccw
  line L42 (127.0355, -21.0355) -> (121.9645, -15.9645)
  arc A34 (120.5, -12.4289) -> (121.9645, -15.9645) centre (125.5, -12.4289) ccw
  line L43 (120.5, -12.4289) -> (120.5, -9.5)
  arc A35 (125.5, -4.5) -> (120.5, -9.5) centre (125.5, -9.5) ccw
  line L44 (5, -11.5) -> (5, -9.5)
  line L45 (56, -38.5) -> (56, -40.5)
  line L46 (5, -9.5) -> (56, -9.5)
  line L47 (56, -9.5) -> (56, -40.5)
  line L48 (56, -40.5) -> (5, -40.5)
  line L49 (5, -40.5) -> (5, -9.5)
  dimension "d151" = 2
  dimension "d152" = 2
  dimension "d153" = 2
  dimension "d154" = 2
  constraint horizontal L46
  constraint vertical L47
  constraint horizontal L48
  constraint vertical L49
  measures "d151" distance of L1.end L44.start
  measures "d152" distance of L44.start L44.end
  measures "d153" distance of L0.start L45.start
  measures "d154" distance of L45.start L45.end
extrude "Extrusion10" cut sketch "Skizze9" against normal blind 3 contours L44 L45 L46 L47 L48 L49
extrude "Extrusion11" add 1 faces at (53.1667, 48.5, 20) along direction (0, 0, 1) blind 5
